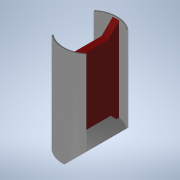
# Autodesk Inventor part: cansat_estructura3
Saved by Autodesk Inventor 2021.3 (Build 253353010, 353A)
## iProperties
Created: 2021-08-20
Part Number: cansat_estructura3
Material: Generic
Document SubType Name: Modeling
Designer: pili2
Density: 1 g/cm^3
Appearance: Default
Author: pili2
Autodesk Inventor part; units mm, degrees
ref_plane "XZ Plane" through (0, 0, 0) normal (0, 1, 0) x (-1, 0, 0)
ref_plane "XY Plane" through (0, 0, 0) normal (0, 0, 1) x (1, 0, 0)
sketch "Sketch1" plane through (0, 0, 0) normal (0, 1, 0) x (-1, 0, 0)
  circle A0 centre (0, 0) radius 33
  dimension "d0" = 66
  constraints: 1 centre point, 1 coincident
  measures "d0" diameter of A0
extrude "Extrusion1" add sketch "Sketch1" along normal blind 121
sketch "Sketch2" plane through (0, 121, 0) normal (0, 1, 0) x (1, 0, 0)
  circle A0 centre (0, 0) radius 31.5
  dimension "d3" = 63
  constraints: 1 centre point, 1 coincident
  measures "d3" diameter of A0
extrude "Extrusion2" cut sketch "Sketch2" against normal blind 103
sketch "Sketch3" plane through (0, 0, 0) normal (1, 0, 0) x (0, 1, 0)
  line L0 (121, 31.5) -> (121, -31.5) projected
  line L1 (0, -33) -> (0, 33) projected
  line L2 (5.9121, 31.5) -> (5.9121, 28)
  line L3 (5.9121, 28) -> (25, 28)
  line L4 (25, 28) -> (25, -28)
  line L5 (25, -28) -> (5.9121, -28)
  line L6 (5.9121, -28) -> (5.9121, -31.5)
  line L7 (121, -33) -> (121, 33) projected
  line L8 (119.5, 31.5) -> (106, 18)
  line L9 (106, 18) -> (106, -18)
  line L10 (106, -18) -> (119.5, -31.5)
  line L11 (121, 31.5) -> (18, 31.5) projected
  line L12 (121, -31.5) -> (18, -31.5) projected
  line L13 (121, 31.5) -> (18, 31.5) projected
  line L14 (119.5, 31.5) -> (5.9121, 31.5)
  line L15 (5.9121, -31.5) -> (119.5, -31.5)
  line L16 (121, -31.5) -> (18, -31.5) projected
  point P0 (5.9121, -33)
  point P1 (25, 0)
  point P2 (121, 0)
  dimension "d13" = 25
  dimension "d17" = 15
  dimension "d19" = 15
  dimension "d33" = 3.5
  constraints: 20 end point, 6 point on line, 4 perpendicular, 2 midpoint, 1 collinear, 1 horizontal alignment, 1 parallel, 1 vertical
  measures "d13" distance between parallel lines of L1 L4
  measures "d17" horizontal distance of L7.end L8.end
  measures "d19" horizontal distance of L9.end L7.start
  measures "d33" distance between parallel lines of L13 L3
extrude "Extrusion4" add sketch "Sketch3" along normal mid plane 8 separate body contours L8 L9 L10 L12 L15 L6 L5 L4 L3 L2 L14 L11
ref_plane "Work Plane1" through (20, 0, 0) normal (1, 0, 0) x (0, 1, 0)
ref_plane "Work Plane2" through (-20, 0, 0) normal (1, 0, 0) x (0, 1, 0)
sketch "Sketch4" plane through (20, 0, 0) normal (1, 0, 0) x (0, 1, 0)
  line L0 (-18.9358, -46.7949) -> (142.2545, -46.7949)
  line L1 (142.2545, -46.7949) -> (142.2545, 56.6765)
  line L2 (142.2545, 56.6765) -> (-18.9358, 56.6765)
  line L3 (-18.9358, 56.6765) -> (-18.9358, -46.7949)
  point P0 (0, 0)
  constraints: 8 end point, 2 parallel, 1 horizontal, 1 perpendicular
extrude "Extrusion5" cut sketch "Sketch4" along normal blind 100 bodies 1
sketch "Sketch5" plane through (-20, 0, 0) normal (1, 0, 0) x (0, 1, 0)
  line L0 (136.7321, -48.8329) -> (-13.7148, -48.8329)
  line L1 (-13.7148, -48.8329) -> (-13.7148, 47.5861)
  line L2 (-13.7148, 47.5861) -> (136.7321, 47.5861)
  line L3 (136.7321, 47.5861) -> (136.7321, -48.8329)
  point P0 (0, 0)
  constraints: 8 end point, 2 parallel, 1 horizontal, 1 perpendicular
extrude "Extrusion6" cut sketch "Sketch5" against normal blind 100 bodies 1
chamfer "Chamfer5" distance 18 angle 45 1 edges at (20, 0, 0)
body "Solid1"
body "Solid2"
